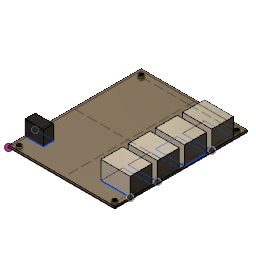
ZodiacFX (Autodesk Fusion 360 design; units mm, degrees)
Autodesk Fusion 360 part; units mm, degrees
sketch "Sketch1" plane through (0, 0, 0) normal (0, 1, 0) x (1, 0, 0)
  line L0 (0, 0) -> (80, 0)
  line L1 (80, 0) -> (80, 100)
  line L2 (80, 100) -> (0, 100)
  line L3 (0, 100) -> (0, 0)
  circle A0 centre (4, 96) radius 1.5
  circle A1 centre (76, 96) radius 1.5
  circle A2 centre (76, 4) radius 1.5
  circle A3 centre (4, 4) radius 1.5
  line L4 (40, 100) -> (40, 0) construction
  line L5 (0, 50) -> (80, 50) construction
  line L6 (4, 96) -> (40, 96) construction
  line L7 (76, 96) -> (76, 50) construction
  line L8 (76, 96) -> (40, 96) construction
  line L9 (76, 50) -> (76, 4) construction
  dimension "d1" = 80
  dimension "d2" = 100
  dimension "d3" = 3
  dimension "d4" = 72
  dimension "d5" = 92
  measures "d1" distance of L0.start
  measures "d3" diameter of A0
  measures "d5" distance of L0.start
extrude "Extrude1" add sketch "Sketch1" along normal blind 1.6
sketch "Sketch2" plane through (0, 1.6, 0) normal (0, 1, 0) x (-1, 0, 0)
  circle A0 centre (-4, -96) radius 1.5
  circle A1 centre (-4, -4) radius 1.5
  circle A2 centre (-76, -96) radius 1.5
  circle A3 centre (-76, -4) radius 1.5
  line L0 (0, -100) -> (0, 0)
  line L1 (0, 0) -> (-80, 0)
  line L2 (-80, 0) -> (-80, -100)
  line L3 (-80, -100) -> (0, -100)
  line L4 (-58, -89.6377) -> (-80, -89.6377)
  line L5 (-80, -89.6377) -> (-80, -73.1377)
  line L6 (-80, -73.1377) -> (-58, -73.1377)
  line L7 (-58, -73.1377) -> (-58, -89.6377)
  line L8 (-58, -69.1377) -> (-80, -69.1377)
  line L9 (-80, -69.1377) -> (-80, -52.6377)
  line L10 (-80, -52.6377) -> (-58, -52.6377)
  line L11 (-58, -52.6377) -> (-58, -69.1377)
  line L12 (-58, -48.6377) -> (-80, -48.6377)
  line L13 (-80, -48.6377) -> (-80, -32.1377)
  line L14 (-80, -32.1377) -> (-58, -32.1377)
  line L15 (-58, -32.1377) -> (-58, -48.6377)
  line L16 (-58, -28.1377) -> (-80, -28.1377)
  line L17 (-80, -28.1377) -> (-80, -11.6377)
  line L18 (-80, -11.6377) -> (-58, -11.6377)
  line L19 (-58, -11.6377) -> (-58, -28.1377)
  line L20 (0, -20) -> (-14.1052, -20)
  line L21 (-14.1052, -20) -> (-14.1052, -12.0995)
  line L22 (-14.1052, -12.0995) -> (0, -12.0995)
  line L23 (0, -12.0995) -> (0, -20)
  dimension "d8" = 16.5
  dimension "d9" = 22
  dimension "d10" = 4
  dimension "d11" = 4
  dimension "d12" = 4
  measures "d10" distance of L6 L8
  measures "d11" distance of L10 L12
  measures "d12" distance of L14 L16
extrude "Extrude2" add sketch "Sketch2" along normal blind 13.8 contours L2 L4 L5 L6 L7 | L2 L8 L9 L10 L11 | L2 L16 L17 L18 L19 | L2 L12 L13 L14 L15
extrude "Extrude3" add sketch "Sketch2" along normal blind 11 contours L0 L20 L21 L22 L23
sketch "Sketch3" plane through (0, 1.6, 0) normal (0, 1, 0) x (-1, 0, 0)
